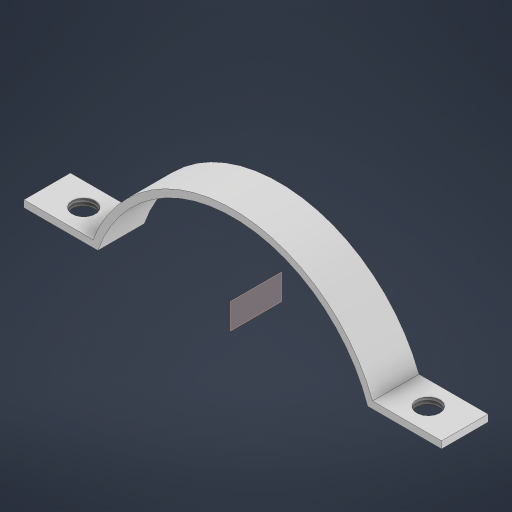
# Autodesk Inventor part: Holder
Saved by Autodesk Inventor 2023 (Build 270158000, 158)
## iProperties
Created: 2022-09-19
Part Number: Holder
Material: Generic
Document SubType Name: Modeling
Designer: Mike
Density: 1 g/cm^3
Appearance: Default
Author: Mike
Autodesk Inventor part; units mm, degrees
ref_plane "YZ Plane" through (0, 0, 0) normal (1, 0, 0) x (0, 1, 0)
ref_plane "XZ Plane" through (0, 0, 0) normal (0, 1, 0) x (-1, 0, 0)
ref_plane "XY Plane" through (0, 0, 0) normal (0, 0, 1) x (1, 0, 0)
sketch "Sketch1" plane through (0, 0, 0) normal (0, 0, 1) x (1, 0, 0)
  arc A0 (58.1571, 20) -> (-58.1571, 20) centre (0, 0) ccw
  line L0 (-90, 0) -> (90, 0) construction
  line L1 (-90, 20) -> (90, 20)
  line L2 (-90, 23) -> (90, 23)
  line L3 (-90, 20) -> (-90, 23)
  line L4 (90, 20) -> (90, 23)
  arc A1 (61.3209, 20) -> (-61.3209, 20) centre (0, 0) ccw
  point P0 (60.2599, 23)
  point P1 (-60.2599, 23)
  dimension "d8" = 123
  dimension "d12" = 90
  dimension "d13" = 90
  dimension "d14" = 0
  dimension "d15" = 20
  dimension "d16" = 3
  dimension "d17" = 129
  dimension "d18" = 180
  dimension "d19" = 90
  constraints: 10 end point, 4 point on circle, 4 point on line, 3 parallel, 2 centre point, 2 coincident, 1 horizontal, 1 vertical
  measures "d8" diameter of A0
  measures "d12" distance of L0.start point (0, 0)
  measures "d13" distance of L0.end point (0, 0)
  measures "d14" distance from line of point (0, 0) L0
  measures "d15" distance between parallel lines of L0 L1
  measures "d16" distance between parallel lines of L1 L2
  measures "d17" diameter of A1
  measures "d18" distance between parallel lines of L4 L3
  measures "d19" distance from line of point (0, 0) L4
extrude "Extrusion2" add sketch "Sketch1" against normal blind 20 contours A0 L2 A1 L1 | A0 L2 A1 | L1 A1 L2 A0 | A1 L2 L4 L1 | L1 L3 L2 A1
sketch "Sketch2" plane through (60.2599, 23, 0) normal (0, 1, 0) x (1, 0, 0)
  circle A0 centre (14, 10) radius 5
  line L0 (29.7401, 0) -> (0, 0) projected
  point P0 (-60.2599, 0)
  dimension "d22" = 10
  dimension "d23" = 10
  dimension "d24" = 14
  constraints: 1 centre point
  measures "d22" distance from line of L0 A0.centre
  measures "d23" diameter of A0
  measures "d24" horizontal distance of L0.end A0.centre
hole "Hole1" at (74.2599, 23, -10) direction (0, -1, 0) diameter 10 end through all
ref_plane "Work Plane1" through (0, 20, 0) normal (1, 0, 0) x (0, 0, -1)
thread "Thread1" size "M10x1.5" class "6H" standard "ANSI Metric M Profile" full length
mirror "Mirror1" about plane through (0, 20, 0) normal (1, 0, 0) of "Hole1"
body "Solid2"
